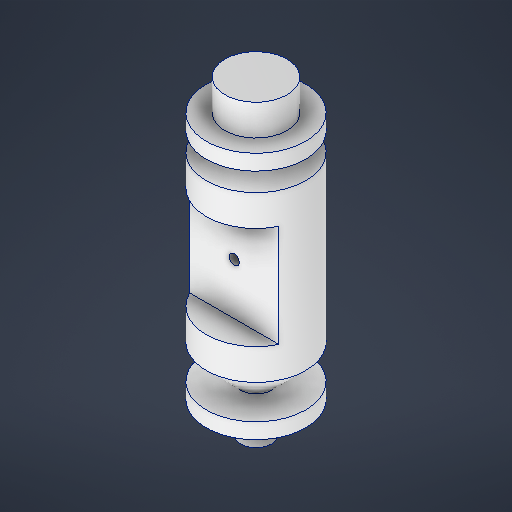
# Autodesk Inventor part: MMAE 232 Assignment 1e-Nicholas Skiba
Saved by Autodesk Inventor 2026.1 (Build 301233000, 233)
## iProperties
Created: 2025-08-26
Part Number: MMAE 232 Assignment 1e-Nicholas Skiba
Material: Aluminum 6061
Document SubType Name: Modeling
Designer: Nick
Density: 2.7 g/cm^3
Appearance: Aluminum - Flat
Mass: 150.347 g
Surface Area: 121.767 cm^2
Volume: 55.6842 cm^3
Author: Nick
Autodesk Inventor part; units mm, degrees
ref_plane "XZ Plane" through (0, 0, 0) normal (0, 1, 0) x (-1, 0, 0)
ref_plane "XY Plane" through (0, 0, 0) normal (0, 0, 1) x (1, 0, 0)
sketch "Sketch1" plane through (0, 0, 0) normal (0, 1, 0) x (-1, 0, 0)
  circle A0 centre (0, 0) radius 16
  dimension "d0" = 32
  constraints: 1 centre point, 1 coincident
  measures "d0" diameter of A0
extrude "Extrusion1" add sketch "Sketch1" along normal blind 70
chamfer "Chamfer1" distance 6 angle 45 1 edges at (16, 70, 0)
chamfer "Chamfer2" distance 11 angle 45 1 edges at (16, 0, 0)
sketch "Sketch2" plane through (0, 70, 0) normal (0, 1, 0) x (1, 0, 0)
  circle A0 centre (0, 0) radius 16
  constraints: 1 centre point, 1 coincident
extrude "Extrusion2" add sketch "Sketch2" along normal blind 5
sketch "Sketch3" plane through (0, 0, 0) normal (0, -1, 0) x (1, 0, 0)
  circle A0 centre (0, 0) radius 16
  constraints: 1 centre point, 1 coincident
extrude "Extrusion3" add sketch "Sketch3" along normal blind 5
sketch "Sketch4" plane through (0, -5, 0) normal (0, -1, 0) x (1, 0, 0)
  circle A0 centre (0, 0) radius 5
  constraints: 1 centre point, 1 coincident
extrude "Extrusion4" add sketch "Sketch4" along normal blind 10
sketch "Sketch5" plane through (0, 75, 0) normal (0, 1, 0) x (1, 0, 0)
  circle A0 centre (0, 0) radius 10
  constraints: 1 centre point, 1 coincident
extrude "Extrusion5" add sketch "Sketch5" along normal blind 10
ref_plane "Work Plane1" through (16, 0, 0) normal (1, 0, 0) x (0, 1, 0)
sketch "Sketch6" plane through (16, 0, 0) normal (1, 0, 0) x (0, 1, 0)
  line L0 (11, 16) -> (11, -16) projected
  line L1 (11, 0) -> (21, 0)
  line L2 (21, 0) -> (21, 7)
  line L3 (11, 16) -> (64, 16) projected
  line L4 (21, 7) -> (54, 7)
  line L5 (54, 7) -> (54, 16)
  line L6 (54, 16) -> (21, 16)
  line L7 (21, 16) -> (21, 7)
  point P0 (0, 0)
  dimension "d17" = 10
  dimension "d18" = 7
  dimension "d19" = 33
  constraints: 12 end point, 2 horizontal, 2 parallel, 2 perpendicular, 1 midpoint, 1 point on line
  measures "d17" distance of L1.start L1.end
  measures "d18" distance of L1.end L2.end
  measures "d19" distance of L6.end L5.end
extrude "Extrusion6" cut sketch "Sketch6" against normal through all contours L3 L5 L4 L7
sketch "Sketch7" plane through (-14.3875, 21, 7) normal (0, 0, 1) x (1, 0, 0)
  line L0 (28.775, 0) -> (0, 0) projected
  line L1 (14.3875, 0) -> (14.3875, 16.5)
  point P0 (14.3875, -21)
  dimension "d22" = 16.5
  constraints: 2 end point, 1 midpoint, 1 vertical
  measures "d22" distance of L1.start L1.end
hole "Hole1" at (0, 37.5, 7) direction (0, 0, -1) diameter 3.242 end through all thread size "M4x0.7" class "6H" standard "ANSI Metric M Profile"
body "Solid1"
